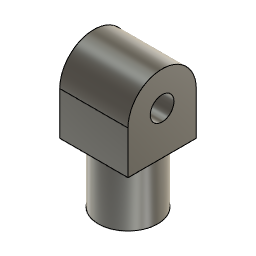
maturita5-phone_holder v2 (Autodesk Fusion 360 design; units mm, degrees)
Autodesk Fusion 360 part; units mm, degrees
note: some values were not read from the file. Set by a fixed rule: which sketch regions a step uses.
sketch "Sketch1" plane through (0, 0, 0) normal (0, 0, 1) x (1, 0, 0)
  circle A0 centre (0, 0) radius 5
  circle A1 centre (0, 0) radius 2.5
  dimension "d1" = 10
  dimension "d2" = 5
  constraint coincident A0.centre A1.centre
  constraint concentric A0 A1
  measures "d1" diameter of A0
  measures "d2" diameter of A1
extrude "Extrude1" add sketch "Sketch1" along normal blind 10
sketch "Sketch2" plane through (0, 0, 10) normal (0, 0, 1) x (-1, 0, 0)
  circle A0 centre (0, 0) radius 2.5
  circle A1 centre (0, 0) radius 5
  line L0 (0, 0) -> (-5.75, 0)
  line L1 (-5.75, 0) -> (-5.75, -5.75)
  line L2 (-5.75, -5.75) -> (5.75, -5.75)
  line L3 (5.75, -5.75) -> (5.75, 5.75)
  line L4 (5.75, 5.75) -> (-5.75, 5.75)
  line L5 (-5.75, 5.75) -> (-5.75, -5.75)
  dimension "d5" = 5.75
  dimension "d6" = 5.75
  dimension "d7" = 11.5
  dimension "d8" = 11.5
  constraint coincident A0.centre A1.centre
  constraint horizontal L0
  constraint perpendicular L0 L1
  constraint horizontal L2
  constraint vertical L3
  constraint horizontal L4
  constraint vertical L5
  measures "d5" distance of A0.centre L0.end
  measures "d6" distance of L0.end L1.end
  measures "d7" distance of L1.end L2.end
  measures "d8" distance of L1.end L4.end
extrude "Extrude2" add sketch "Sketch2" along normal blind 13 contours A0 | A1 | L1 L2 L3 L4 L5
fillet "Fillet1" radius 5.75 2 edges at (0, -5.75, 23) (0, 5.75, 23)
hole "Hole1" at (5.75, 0, 17.25) direction (-1, 0, 0) diameter 4 depth 11.5 tip angle 180
equation "d5 = ( 11.5 / 2 ) * 1 mm"
